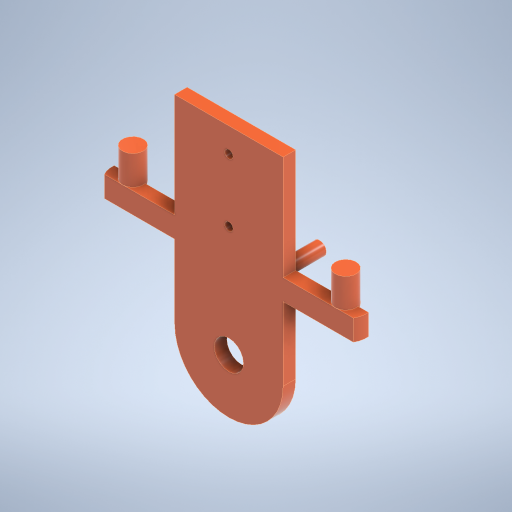
# Autodesk Inventor part: pintutucu
Saved by Autodesk Inventor 2023.2 (Build 272271000, 271)
## iProperties
Created: 2022-11-27
Part Number: pintutucu
Material: Generic
Document SubType Name: Modeling
Designer: omrfrkmll
Density: 1 g/cm^3
Appearance: Smooth - Light Orange
Author: omrfrkmll
Autodesk Inventor part; units mm, degrees
ref_plane "YZ Plane" through (0, 0, 0) normal (1, 0, 0) x (0, 1, 0)
ref_plane "XZ Plane" through (0, 0, 0) normal (0, 1, 0) x (-1, 0, 0)
ref_plane "XY Plane" through (0, 0, 0) normal (0, 0, 1) x (1, 0, 0)
sketch "Sketch1" plane through (0, 0, 0) normal (0, 0, 1) x (1, 0, 0)
  line L0 (0, 8.9678) -> (0, -21.984)
  line L1 (-55.9342, 0) -> (8.6032, 0)
  circle A0 centre (-8.75, 0) radius 1.6
  circle A1 centre (8.75, 0) radius 1.6
  line L2 (-13, 27.4955) -> (13, 27.4955)
  line L3 (13, 27.4955) -> (13, -20.0499)
  line L4 (-13, -20.0499) -> (-13, 27.4955)
  circle A2 centre (0, 21.5844) radius 1
  circle A3 centre (0, 6.5844) radius 1
  circle A4 centre (0, -20.0499) radius 3.5
  line L5 (0, -20.0499) -> (8.75, 0)
  arc A5 (-13, -20.0499) -> (13, -20.0499) centre (0, -20.0499) ccw
  line L6 (-13, 2.4955) -> (-33, 2.4955)
  line L7 (-33, 2.4955) -> (-33, -2.5045)
  line L8 (-33, -2.5045) -> (-13, -2.5045)
  line L9 (13, 2.4955) -> (33, 2.4955)
  line L10 (33, 2.4955) -> (33, -2.5045)
  line L11 (33, -2.5045) -> (13, -2.5045)
  point P0 (0, 0)
  point P1 (-13, -2.5045)
  dimension "d1" = 17.5
  dimension "d2" = 3.2
  dimension "d3" = 15
  dimension "d4" = 2
  dimension "d7" = 26
  dimension "d8" = 7
  dimension "d9" = 21.876
  dimension "d14" = 5
  dimension "d15" = 20
  dimension "d22" = 25
  constraints: 24 end point, 6 centre point, 6 point on line, 5 horizontal, 4 symmetric about line, 2 equal radius, 2 parallel, 2 perpendicular, 2 point on circle, 2 vertical, 1 tangent, 3 other
  measures "d1" distance of A0.centre L5.end
  measures "d2" diameter of A1
  measures "d3" distance of A3.centre A2.centre
  measures "d4" diameter of A2
  measures "d7" distance between parallel lines of L3 L4
  measures "d8" diameter of A4
  measures "d9" distance of L5.start L5.end
  measures "d14" distance between parallel lines of L8 L6
  measures "d15" distance between parallel lines of L4 L7
  measures "d22" distance between parallel lines of L6 L2
extrude "Extrusion1" add sketch "Sketch1" along normal blind 3 contours L1 A1 L5 A4 L0 | L7 L6 L4 L1 | L1 L4 L8 L7 | L4 L2 L3 A5 | L3 L9 L10 L11
sketch "Sketch2" plane through (0, 0, 0) normal (0, 0, -1) x (-1, 0, 0)
  circle A0 centre (-8.75, 0) radius 1.6 projected
  circle A1 centre (-8.75, 0) radius 1.6
  circle A2 centre (8.75, 0) radius 1.6 projected
  circle A3 centre (8.75, 0) radius 1.6
  point P0 (0, 0)
  constraints: 2 centre point, 2 coincident
extrude "Extrusion2" add sketch "Sketch2" along normal blind 10 and the other way blind 3
sketch "Sketch3" plane through (-33, 2.4955, 0) normal (0, 1, 0) x (1, 0, 0)
  circle A0 centre (7.5, -0.5) radius 2.5
  line L0 (20, 0) -> (0, 0) projected
  line L1 (0, 0) -> (0, -3) projected
  line L2 (0.0505, -3) -> (0, -3)
  line L3 (0, -3) -> (0, 0)
  line L4 (0, 0) -> (9.9495, 0)
  line L5 (20, -3) -> (0, -3) projected
  point P0 (33, 0)
  point P1 (5.1646, -1.3921)
  dimension "d16" = 5
  dimension "d26" = 7.5
  constraints: 6 end point, 2 point on circle, 1 centre point, 1 horizontal, 1 perpendicular, 1 point on line, 1 tangent
  measures "d16" diameter of A0
  measures "d26" distance from line of A0.centre L1
extrude "Extrusion3" add sketch "Sketch3" along normal blind 7 contours A0 L0 | L0 A0
fillet "Fillet1" radius 2 2 edges at (10.35, 0, 0) (-7.15, 0, 0)
fillet "Fillet2" radius 1.9 1 edges at (-25.5, 2.4955, 0)
mirror "Mirror1" about plane through (0, 0, 0) normal (1, 0, 0) of "Extrusion3"
mirror "Mirror3" about plane through (0, 0, 0) normal (1, 0, 0) of "Fillet2"
sketch "Sketch5" plane through (25.5, 9.4955, 0.5) normal (0, 1, 0) x (1, 0, 0)
  circle A0 centre (0, 0) radius 5
  line L0 (-12.5, -2.5) -> (7.5, -2.5) projected
  line L1 (4.3301, -2.5) -> (9.1307, -2.5)
  line L2 (9.1307, -2.5) -> (9.1307, 0.5)
  line L3 (9.1307, 0.5) -> (4.9749, 0.5)
  line L4 (-12.5, 0.5) -> (7.5, 0.5) projected
  point P0 (-25.5, 0.5)
  dimension "d27" = 10
  constraints: 6 end point, 2 point on circle, 2 point on line, 1 centre point, 1 horizontal, 1 perpendicular
  measures "d27" diameter of A0
extrude "Extrusion5" cut sketch "Sketch5" against normal up to surface (12 mm away) contours A0 L3 L2 L1 L0
mirror "Mirror4" about plane through (0, 0, 0) normal (1, 0, 0) of "Extrusion5"
body "Solid1"
